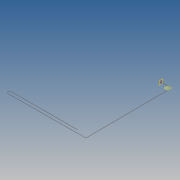
# Autodesk Inventor part: Seil-3
Saved by Autodesk Inventor 2015 SP1 (Build 190203100, 203)
## iProperties
Created: 2015-03-05
Part Number: Seil-3
Material: Generisch
Document SubType Name: Modeling
Designer: Marc
Density: 1 g/cm^3
Appearance: Vorgabe
Author: Marc
Autodesk Inventor part; units mm, degrees
ref_plane "YZ Plane" through (0, 0, 0) normal (1, 0, 0) x (0, 1, 0)
ref_plane "XZ Plane" through (0, 0, 0) normal (0, 1, 0) x (-1, 0, 0)
ref_plane "XY Plane" through (0, 0, 0) normal (0, 0, 1) x (1, 0, 0)
ref_plane "Arbeitsebene1" through (0, 0, 0) normal (0, 0, 1) x (1, 0, 0)
sketch "Skizze1" plane through (0, 0, 0) normal (0, 0, 1) x (1, 0, 0)
  circle A0 centre (0, 0) radius 10 projected
  circle A1 centre (3.435, -479.9877) radius 10 projected
  circle A2 centre (-436.5537, -483.1365) radius 10 projected
  line L0 (0, 10) -> (-50.5578, 10)
  line L1 (9.9997, 0.0716) -> (13.4348, -479.9161)
  line L2 (3.435, -489.9877) -> (-436.4822, -493.1362)
  line L3 (-436.4822, -473.1367) -> (-52.6532, -473.1367)
  arc A3 (9.9997, 0.0716) -> (0, 10) centre (0, 0) ccw
  arc A4 (3.435, -489.9877) -> (13.4348, -479.9161) centre (3.435, -479.9877) ccw
  arc A5 (-436.4822, -473.1367) -> (-436.4822, -493.1362) centre (-436.5537, -483.1365) ccw
  point P0 (0, 0)
  constraints: 12 point on circle, 8 end point, 5 tangent, 3 centre point, 3 concentric, 2 horizontal
ref_plane "Arbeitsebene2" through (-50.5578, 10, 0) normal (-1, 0, 0) x (0, -1, 0)
sketch "Skizze2" plane through (-50.5578, 10, 0) normal (-1, 0, 0) x (0, -1, 0)
  circle A0 centre (0, 0) radius 1
  point P0 (10, 0)
  dimension "d0" = 2
  constraints: 1 centre point, 1 coincident
  measures "d0" diameter of A0
sweep "Sweeping1" add profiles "Skizze2" path "Skizze1" path curves L0 A3 L1 A4 L2 A5 L3
